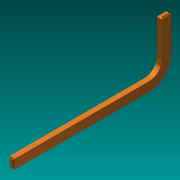
# Autodesk Inventor part: PinRight2
Saved by Autodesk Inventor 2015 (Build 190159000, 159)
## iProperties
Created: 2014-07-19
Part Number: PinRight2
Material: Gold
Document SubType Name: Modeling
Designer: Sawaiz Syed
Density: 19.3 g/cm^3
Appearance: Metal 1600F Hot
Author: Sawaiz Syed
Autodesk Inventor part; units mm, degrees
note: some values were not read from the file. Chosen so that the rebuilt part matches the saved one: bend side of "Bend Part1".
ref_plane "YZ Plane" through (0, 0, 0) normal (1, 0, 0) x (0, 1, 0)
ref_plane "XZ Plane" through (0, 0, 0) normal (0, 1, 0) x (-1, 0, 0)
ref_plane "XY Plane" through (0, 0, 0) normal (0, 0, 1) x (1, 0, 0)
sketch "Sketch1" plane through (0, 0, 0) normal (0, 1, 0) x (-1, 0, 0)
  line L0 (0.2032, -0.381) -> (-0.2032, -0.381)
  line L1 (-0.2032, -0.381) -> (-0.2032, 0.381)
  line L2 (-0.2032, 0.381) -> (0.2032, 0.381)
  line L3 (0.2032, 0.381) -> (0.2032, -0.381)
  line L4 (0.2032, -0.381) -> (-0.2032, 0.381) construction
  line L5 (-0.2032, -0.381) -> (0.2032, 0.381) construction
  point P0 (0, 0)
  dimension "d0" = 0.4064
  dimension "d1" = 0.762
  constraints: 12 end point, 2 midpoint, 2 parallel, 1 horizontal, 1 perpendicular
  measures "d0" distance of L1.end L2.end
  measures "d1" distance of L0.end L1.end
extrude "Extrusion1" add sketch "Sketch1" along normal blind 15.4
chamfer "Chamfer1" distance 0.1 angle 45 8 edges at (0.2032, 15.4, 0) (0, 15.4, -0.381) (0, 15.4, 0.381) (-0.2032, 15.4, 0) (0.2032, 0, 0) (0, 0, -0.381) (0, 0, 0.381) (-0.2032, 0, 0)
sketch "Sketch2" plane through (-0.2032, 0.1, 0.381) normal (0, 0, 1) x (1, 0, 0)
  line L0 (-1.0405, 10.84) -> (1.7368, 10.84)
  point P0 (0.2032, -0.1)
  dimension "d7" = 10.94
  constraints: 2 end point, 1 horizontal
  measures "d7" distance from line of point (0.203, -0.1) L0
bend part "Bend Part1" radius 1 angle 90 line through (-1.2437, 10.94, 0.381) along (1, 0, 0) centre toward (0, 0, 1) moving side (0, 1, 0) both sides no
body "Solid1"
